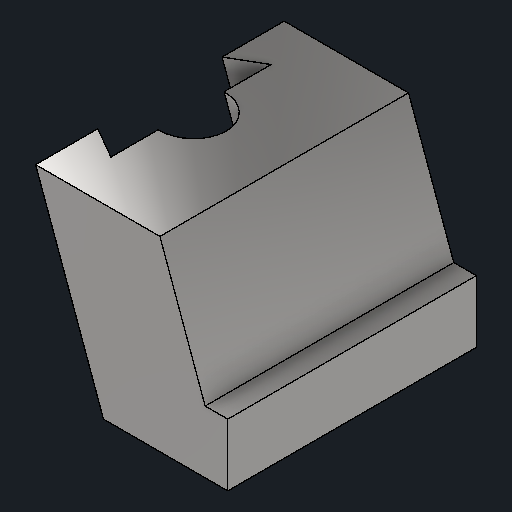
# Autodesk Inventor part: Part1
Saved by Autodesk Inventor 2026.2 (Build 302298000, 298)
## iProperties
Created: 2026-09-23
Part Number: Part1
Material: Steel, Alloy
Document SubType Name: Modeling
Designer: JoshuaEah
Density: 7.73 g/cm^3
Appearance: Semi-Polished
Author: JoshuaEah
Autodesk Inventor part; units mm, degrees
ref_plane "YZ Plane" through (0, 0, 0) normal (1, 0, 0) x (0, 1, 0)
ref_plane "XZ Plane" through (0, 0, 0) normal (0, 1, 0) x (-1, 0, 0)
sketch "Sketch1" plane through (0, 0, 0) normal (0, 1, 0) x (-1, 0, 0)
  line L0 (0, 0) -> (-12.7, 0)
  line L1 (-12.7, 0) -> (-12.7, -25.4)
  line L2 (-12.7, -25.4) -> (0, -25.4)
  line L3 (0, -25.4) -> (0, 0)
  line L4 (0, -12.7) -> (-12.7, -12.7) construction
  line L5 (-3.175, -25.4) -> (-3.175, 0)
  line L6 (-3.175, -20.8831) -> (0, -19.05)
  line L7 (-3.175, -4.5169) -> (0, -6.35)
  line L8 (-9.525, -25.4) -> (-9.525, 0)
  point P0 (-3.175, -12.7)
  point P1 (0, -6.35)
  dimension "d0" = 12.7
  dimension "d7" = 25.4
  dimension "d34" = 3.175
  dimension "d35" = 60
  dimension "d36" = 12.7
  dimension "d57" = 3.175
  constraints: 18 end point, 6 point on line, 3 midpoint, 3 perpendicular, 2 parallel, 2 symmetric about line, 1 coincident, 1 horizontal
  measures "d0" distance of L2.end L1.end
  measures "d7" distance of L2.end L0.start
  measures "d34" distance between parallel lines of L3 L5
  measures "d35" angle of L3 L6
  measures "d36" diameter of L6.end L4
  measures "d57" distance between parallel lines of L1 L8
sketch "Sketch8" plane through (0, 0, 0) normal (0, 0, 1) x (1, 0, 0)
  line L0 (0, 0) -> (-6.9336, 19.05)
  line L1 (0, 0) -> (20.2726, 0) construction
  dimension "d53" = 110
  dimension "d54" = 19.05
  constraints: 4 end point, 1 coincident, 1 equal length, 1 horizontal
  measures "d53" angle of L1 L0
  measures "d54" distance from line of L1 L0.end
sweep "Sweep3" add profiles "Sketch1" path "Sketch8" contours L3 L7 L5 L0 | L5 L2 L8 L0 | L8 L2 L1 L0 | L3 L2 L5 L6
extrude "Extrusion3" add sketch "Sketch1" along normal blind 6.35 contours L8 L2 L1 L0
ref_plane "Work Plane6" through (-3.7586, 19.05, -25.4) normal (-0.342, 0.9397, 0) x (0, 0, 1)
sketch "Sketch9" plane through (-3.7586, 19.05, -25.4) normal (-0.342, 0.9397, 0) x (0, 0, 1)
  line L0 (4.5169, 0) -> (20.8831, 0) construction
  point P0 (12.7, 0)
  constraints: 1 midpoint
hole "Hole4" at (-3.7586, 19.05, -12.7) direction (0.342, -0.9397, 0) diameter 6.7564 depth 12.7 tip angle 118
equation "\"slopeAngle\" = 70deg"
body "Solid4"
